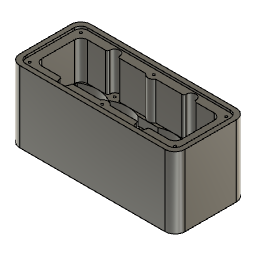
Main Clock Body (Autodesk Fusion 360 design; units mm, degrees)
Autodesk Fusion 360 part; units mm, degrees
sketch "Main Body" plane through (0, 0, 0) normal (0, 0, 1) x (1, 0, 0)
  line L0 (51, 25) -> (-51, 25)
  line L1 (-58, 18) -> (-58, -18)
  line L2 (-51, -25) -> (51, -25)
  line L3 (58, -18) -> (58, 18)
  line L4 (58, 25) -> (-58, -25) construction
  line L5 (-58, 25) -> (58, -25) construction
  arc A0 (-51, 25) -> (-58, 18) centre (-51, 18) ccw
  arc A1 (-58, -18) -> (-51, -25) centre (-51, -18) ccw
  arc A2 (51, -25) -> (58, -18) centre (51, -18) ccw
  arc A3 (58, 18) -> (51, 25) centre (51, 18) ccw
  line L6 (-50, -21.8) -> (50, -21.8)
  line L7 (-54.8, -21.8) -> (54.8, 21.8) construction
  line L8 (54.8, -21.8) -> (-54.8, 21.8) construction
  line L9 (-50, -21.8) -> (50, -21.8)
  line L10 (-50, -21.8) -> (50, -21.8)
  dimension "d1" = 116
  dimension "d2" = 50
  dimension "d3" = 7
  dimension "d4" = 7
  dimension "d5" = 7
  dimension "d6" = 7
  constraint perpendicular L0 L1
  constraint parallel L0 L2
  constraint parallel L1 L3
  constraint horizontal L0
  constraint coincident L4 origin
  constraint coincident L5 origin
  constraint coincident L5.start L0
  constraint coincident L5.start L1
  constraint tangent L0 A0
  constraint tangent L1 A0
  constraint coincident L4.end L1
  constraint coincident L4.end L2
  constraint tangent L1 A1
  constraint tangent L2 A1
  constraint coincident L5.end L2
  constraint coincident L5.end L3
  constraint tangent L2 A2
  constraint tangent L3 A2
  constraint coincident L4.start L3
  constraint coincident L4.start L0
  constraint tangent L3 A3
  constraint tangent L0 A3
  measures "d1" distance of L4.end L5.end
  measures "d2" distance of L5.start L4.end
  measures "d3" radius of A0
  measures "d4" radius of A1
  measures "d5" radius of A2
  measures "d6" radius of A3
  measures "d10" distance of L8.start
extrude "Extrude1" add sketch "Main Body" along normal blind 50
sketch "Back Panel" plane through (0, 0, 50) normal (0, 0, 1) x (-1, 0, 0)
  arc A0 (-58, -18) -> (-51, -25) centre (-51, -18) ccw
  line L0 (-51, -25) -> (51, -25)
  arc A1 (51, -25) -> (58, -18) centre (51, -18) ccw
  line L1 (58, -18) -> (58, 18)
  arc A2 (58, 18) -> (51, 25) centre (51, 18) ccw
  line L2 (51, 25) -> (-51, 25)
  arc A3 (-51, 25) -> (-58, 18) centre (-51, 18) ccw
  line L3 (-58, 18) -> (-58, -18)
  line L4 (-50, -21.8) -> (50, -21.8)
  line L5 (54.8, -17) -> (54.8, 17)
  line L6 (50, 21.8) -> (-50, 21.8)
  line L7 (-54.8, 17) -> (-54.8, -17)
  line L8 (-54.8, -21.8) -> (54.8, 21.8) construction
  line L9 (54.8, -21.8) -> (-54.8, 21.8) construction
  arc A4 (50, -21.8) -> (54.8, -17) centre (50, -17) ccw
  arc A5 (54.8, 17) -> (50, 21.8) centre (50, 17) ccw
  arc A6 (-50, 21.8) -> (-54.8, 17) centre (-50, 17) ccw
  arc A7 (-54.8, -17) -> (-50, -21.8) centre (-50, -17) ccw
  dimension "d9" = 109.6
  dimension "d10" = 43.6
  dimension "d11" = 4.8
  dimension "d12" = 4.8
  dimension "d13" = 4.8
  dimension "d14" = 4.8
  constraint perpendicular L4 L5
  constraint parallel L4 L6
  constraint parallel L5 L7
  constraint horizontal L4
  constraint coincident L8 origin
  constraint coincident L9 origin
  constraint coincident L9.start L4
  constraint coincident L9.start L5
  constraint tangent L4 A4
  constraint tangent L5 A4
  constraint coincident L8.end L5
  constraint coincident L8.end L6
  constraint tangent L5 A5
  constraint tangent L6 A5
  constraint coincident L9.end L6
  constraint coincident L9.end L7
  constraint tangent L6 A6
  constraint tangent L7 A6
  constraint coincident L8.start L7
  constraint coincident L8.start L4
  constraint tangent L7 A7
  constraint tangent L4 A7
  measures "d9" distance of L8.end L9.end
  measures "d10" distance of L9.start L8.end
  measures "d11" radius of A4
  measures "d12" radius of A5
  measures "d13" radius of A6
  measures "d14" radius of A7
extrude "Extrude2" cut sketch "Back Panel" against normal blind 1.6 contours L4 L5 L6 L7 A4 A5 A6 A7
sketch "Electronics Cavity" plane through (0, 0, 48.4) normal (0, 0, 1) x (-1, 0, 0)
  arc A0 (-54.8, -17) -> (-50, -21.8) centre (-50, -17) ccw
  line L0 (-50, -21.8) -> (50, -21.8)
  arc A1 (50, -21.8) -> (54.8, -17) centre (50, -17) ccw
  line L1 (54.8, -17) -> (54.8, 17)
  arc A2 (54.8, 17) -> (50, 21.8) centre (50, 17) ccw
  line L2 (50, 21.8) -> (-50, 21.8)
  arc A3 (-50, 21.8) -> (-54.8, 17) centre (-50, 17) ccw
  line L3 (-54.8, 17) -> (-54.8, -17)
  line L4 (49, 11.5) -> (49, -11.5)
  line L5 (-49, -11.5) -> (-49, 11.5)
  arc A4 (44.5, -16) -> (49, -11.5) centre (44.5, -11.5) ccw
  arc A5 (49, 11.5) -> (44.5, 16) centre (44.5, 11.5) ccw
  arc A6 (-44.5, 16) -> (-49, 11.5) centre (-44.5, 11.5) ccw
  arc A7 (-49, -11.5) -> (-44.5, -16) centre (-44.5, -11.5) ccw
  line L6 (44.5, -16) -> (31.75, -16)
  line L7 (-31.75, -16) -> (-44.5, -16)
  line L8 (31.75, 16) -> (44.5, 16)
  line L9 (-44.5, 16) -> (-31.75, 16)
  arc A8 (-3.4641, 16) -> (3.4641, 16) centre (0, 18) ccw
  line L10 (-3.4641, -16) -> (-21.75, -16)
  line L11 (-21.75, 16) -> (-3.4641, 16)
  line L12 (3.4641, 16) -> (21.75, 16)
  line L13 (26.75, 0) -> (-26.75, 0) construction
  line L14 (26.75, -17.5) -> (26.75, 17.5) construction
  line L15 (-26.75, -17.5) -> (-26.75, 17.5) construction
  line L16 (0, 18) -> (0, -18) construction
  arc A9 (3.4641, -16) -> (-3.4641, -16) centre (0, -18) ccw
  line L17 (49, 0) -> (-49, 0) construction
  arc A10 (23.25, -17.5) -> (30.25, -17.5) centre (26.75, -17.5) ccw
  line L18 (26.75, -17.5) -> (23.25, -17.5) construction
  line L19 (26.75, -17.5) -> (30.25, -17.5) construction
  arc A11 (31.75, -16) -> (30.25, -17.5) centre (31.75, -17.5) ccw
  line L20 (31.75, -17.5) -> (31.75, -16) construction
  line L21 (31.75, -17.5) -> (30.25, -17.5) construction
  line L22 (21.75, -16) -> (3.4641, -16)
  arc A12 (23.25, -17.5) -> (21.75, -16) centre (21.75, -17.5) ccw
  line L23 (21.75, -17.5) -> (23.25, -17.5) construction
  line L24 (21.75, -17.5) -> (21.75, -16) construction
  arc A13 (30.25, 17.5) -> (23.25, 17.5) centre (26.75, 17.5) ccw
  line L25 (26.75, 17.5) -> (30.25, 17.5) construction
  line L26 (26.75, 17.5) -> (23.25, 17.5) construction
  arc A14 (30.25, 17.5) -> (31.75, 16) centre (31.75, 17.5) ccw
  line L27 (31.75, 17.5) -> (30.25, 17.5) construction
  line L28 (31.75, 17.5) -> (31.75, 16) construction
  arc A15 (21.75, 16) -> (23.25, 17.5) centre (21.75, 17.5) ccw
  line L29 (21.75, 17.5) -> (21.75, 16) construction
  line L30 (21.75, 17.5) -> (23.25, 17.5) construction
  arc A16 (-23.25, 17.5) -> (-30.25, 17.5) centre (-26.75, 17.5) ccw
  line L31 (-26.75, 17.5) -> (-23.25, 17.5) construction
  line L32 (-26.75, 17.5) -> (-30.25, 17.5) construction
  arc A17 (-23.25, 17.5) -> (-21.75, 16) centre (-21.75, 17.5) ccw
  line L33 (-21.75, 17.5) -> (-23.25, 17.5) construction
  line L34 (-21.75, 17.5) -> (-21.75, 16) construction
  arc A18 (-31.75, 16) -> (-30.25, 17.5) centre (-31.75, 17.5) ccw
  line L35 (-31.75, 17.5) -> (-31.75, 16) construction
  line L36 (-31.75, 17.5) -> (-30.25, 17.5) construction
  arc A19 (-30.25, -17.5) -> (-23.25, -17.5) centre (-26.75, -17.5) ccw
  line L37 (-26.75, -17.5) -> (-30.25, -17.5) construction
  line L38 (-26.75, -17.5) -> (-23.25, -17.5) construction
  arc A20 (-21.75, -16) -> (-23.25, -17.5) centre (-21.75, -17.5) ccw
  line L39 (-21.75, -17.5) -> (-21.75, -16) construction
  line L40 (-21.75, -17.5) -> (-23.25, -17.5) construction
  arc A21 (-30.25, -17.5) -> (-31.75, -16) centre (-31.75, -17.5) ccw
  line L41 (-31.75, -17.5) -> (-30.25, -17.5) construction
  line L42 (-31.75, -17.5) -> (-31.75, -16) construction
  dimension "d19" = 4.5
  dimension "d20" = 4.5
  dimension "d21" = 4.5
  dimension "d22" = 4.5
  dimension "d52" = 4
  dimension "d99" = 53.5
  dimension "d102" = 36
  dimension "d103" = 4
  dimension "d104" = 98
  dimension "d106" = 32
  dimension "d109" = 35
  dimension "d110" = 3.5
  dimension "d111" = 180
  dimension "d112" = 90
  dimension "d113" = 90
  dimension "d114" = 3.5
  dimension "d115" = 180
  dimension "d116" = 90
  dimension "d117" = 90
  dimension "d118" = 35
  dimension "d119" = 3.5
  dimension "d120" = 180
  dimension "d121" = 90
  dimension "d122" = 90
  dimension "d123" = 3.5
  dimension "d124" = 180
  dimension "d125" = 90
  dimension "d126" = 90
  constraint parallel L6 L9
  constraint parallel L4 L5
  constraint horizontal L9
  constraint tangent A4 L6
  constraint tangent L4 A4
  constraint tangent A5 L9
  constraint tangent L4 A5
  constraint tangent A6 L9
  constraint tangent L5 A6
  constraint tangent L5 A7
  constraint tangent A7 L6
  constraint coincident L8.start L9
  constraint collinear L8 L9
  constraint coincident L11.start L9
  constraint collinear L9 L11
  constraint coincident A8.end L11
  constraint collinear L11 L12
  constraint horizontal L13
  constraint midpoint origin L13
  constraint vertical L14
  constraint midpoint L13.start L14
  constraint vertical L15
  constraint midpoint L13.end L15
  constraint vertical L16
  constraint midpoint origin L16
  constraint coincident L16.end A9.centre
  constraint coincident L10.start A9.end
  constraint horizontal L17
  constraint midpoint origin L17
  constraint coincident L4 L17.start
  constraint coincident L5 L17.end
  constraint vertical L4
  constraint midpoint L4 L17.start
  constraint coincident A8.centre L16.start
  constraint coincident L14.start A10.centre
  constraint horizontal L19
  constraint horizontal L21
  constraint coincident L6.end A11.start
  constraint horizontal L22
  constraint horizontal L23
  constraint coincident L22.start A12.end
  constraint collinear L6 L22
  constraint coincident A9.start L22.end
  constraint coincident L14.end A13.centre
  constraint horizontal L26
  constraint horizontal L27
  constraint coincident L8.start A14.end
  constraint horizontal L30
  constraint coincident L12.end A15.start
  constraint coincident L15.end A16.centre
  constraint horizontal L31
  constraint horizontal L33
  constraint coincident L11.start A17.end
  constraint horizontal L36
  constraint coincident L9.end A18.start
  constraint coincident L15.start A19.centre
  constraint horizontal L38
  constraint horizontal L40
  constraint coincident L10.end A20.start
  constraint collinear L10 L22
  constraint horizontal L41
  constraint coincident L7.start A21.end
  constraint collinear L7 L10
  measures "d19" radius of A4
  measures "d20" radius of A5
  measures "d21" radius of A6
  measures "d22" radius of A7
  measures "d52" radius of A8
  measures "d99" distance of L13.start L13.end
  measures "d102" distance of A8.centre L16.end
  measures "d103" radius of A9
  measures "d104" distance of L17.start L17.end
  measures "d106" distance of A4.start A5.end
  measures "d109" distance of L14.start L14.end
  measures "d110" radius of A10
  measures "d111" angle of L18 L19
  measures "d112" angle of L20 L21
  measures "d113" angle of L23 L24
  measures "d114" radius of A13
  measures "d115" angle of L25 L26
  measures "d116" angle of L27 L28
  measures "d117" angle of L29 L30
  measures "d118" distance of L15.start L15.end
  measures "d119" radius of A16
  measures "d120" angle of L31 L32
  measures "d121" angle of L33 L34
  measures "d122" angle of L35 L36
  measures "d123" radius of A19
  measures "d124" angle of L37 L38
  measures "d125" angle of L39 L40
  measures "d126" angle of L41 L42
extrude "Extrude3" cut sketch "Electronics Cavity" against normal blind 26.6 contours L4 L5 A4 A5 A6 A7 L6 L7 L8 L9 A8 L10 L11 L12 A9 A10 A11 L22 A12 A13 A14 A15 A16 A17 A18 A19 A20 A21
sketch "Tube Cavities" plane through (0, 0, 21.8) normal (0, 0, 1) x (-1, 0, 0)
  line L0 (-31.75, 16) -> (-44.5, 16)
  arc A0 (-44.5, 16) -> (-49, 11.5) centre (-44.5, 11.5) ccw
  line L1 (-49, 11.5) -> (-49, -11.5)
  arc A1 (-49, -11.5) -> (-44.5, -16) centre (-44.5, -11.5) ccw
  line L2 (-44.5, -16) -> (-31.75, -16)
  line L3 (31.75, -16) -> (44.5, -16)
  arc A2 (44.5, -16) -> (49, -11.5) centre (44.5, -11.5) ccw
  line L4 (49, -11.5) -> (49, 11.5)
  arc A3 (49, 11.5) -> (44.5, 16) centre (44.5, 11.5) ccw
  line L5 (44.5, 16) -> (31.75, 16)
  line L6 (21.75, 16) -> (3.4641, 16)
  arc A4 (-3.4641, 16) -> (3.4641, 16) centre (0, 18) ccw
  line L7 (16, 0) -> (-16, 0) construction
  line L8 (37.5, 0) -> (-37.5, 0) construction
  line L9 (37.5, -5) -> (37.5, 5) construction
  arc A5 (48.5, 12.8885) -> (27.25, 13.3286) centre (37.5, -5) ccw
  arc A6 (27.25, -13.3286) -> (48.5, -12.8885) centre (37.5, 5) ccw
  line L10 (37.5, -16) -> (37.5, 16) construction
  line L11 (16, -16) -> (16, 16) construction
  line L12 (16, 5) -> (16, -5) construction
  line L13 (37.5, 0) -> (48.5, 0) construction
  line L14 (48.5, -12.8885) -> (48.5, 12.8885)
  line L15 (27.25, -13.3286) -> (26.25, -13.3286)
  line L16 (27.25, 13.3286) -> (26.25, 13.3286)
  arc A7 (5, -12.8885) -> (26.25, -13.3286) centre (16, 5) ccw
  arc A8 (26.25, 13.3286) -> (5, 12.8885) centre (16, -5) ccw
  line L17 (5, -12.8885) -> (5, 12.8885)
  line L18 (16, 0) -> (5, 0) construction
  line L19 (-16, -5) -> (-16, 5) construction
  line L20 (-16, -16) -> (-16, 16) construction
  line L21 (-16, 0) -> (-5, 0) construction
  line L22 (-37.5, -5) -> (-37.5, 5) construction
  line L23 (-37.5, -16) -> (-37.5, 16) construction
  arc A9 (-48.5, -12.8885) -> (-27.25, -13.3286) centre (-37.5, 5) ccw
  arc A10 (-26.25, -13.3286) -> (-5, -12.8885) centre (-16, 5) ccw
  arc A11 (-5, 12.8885) -> (-26.25, 13.3286) centre (-16, -5) ccw
  arc A12 (-27.25, 13.3286) -> (-48.5, 12.8885) centre (-37.5, -5) ccw
  line L24 (-5, -12.8885) -> (-5, 12.8885)
  line L25 (-48.5, -12.8885) -> (-48.5, 12.8885)
  line L26 (-26.25, -13.3286) -> (-27.25, -13.3286)
  line L27 (-26.25, 13.3286) -> (-27.25, 13.3286)
  line L28 (-37.5, 0) -> (-48.5, 0) construction
  arc A13 (3.4641, -16) -> (-3.4641, -16) centre (0, -18) ccw
  arc A14 (23.25, -17.5) -> (30.25, -17.5) centre (26.75, -17.5) ccw
  arc A15 (31.75, -16) -> (30.25, -17.5) centre (31.75, -17.5) ccw
  arc A16 (30.25, 17.5) -> (31.75, 16) centre (31.75, 17.5) ccw
  arc A17 (30.25, 17.5) -> (23.25, 17.5) centre (26.75, 17.5) ccw
  arc A18 (21.75, 16) -> (23.25, 17.5) centre (21.75, 17.5) ccw
  line L29 (-3.4641, 16) -> (-21.75, 16)
  arc A19 (-23.25, 17.5) -> (-21.75, 16) centre (-21.75, 17.5) ccw
  arc A20 (-23.25, 17.5) -> (-30.25, 17.5) centre (-26.75, 17.5) ccw
  arc A21 (-31.75, 16) -> (-30.25, 17.5) centre (-31.75, 17.5) ccw
  arc A22 (-30.25, -17.5) -> (-31.75, -16) centre (-31.75, -17.5) ccw
  arc A23 (-30.25, -17.5) -> (-23.25, -17.5) centre (-26.75, -17.5) ccw
  arc A24 (-21.75, -16) -> (-23.25, -17.5) centre (-21.75, -17.5) ccw
  line L30 (-21.75, -16) -> (-3.4641, -16)
  line L31 (3.4641, -16) -> (21.75, -16)
  arc A25 (23.25, -17.5) -> (21.75, -16) centre (21.75, -17.5) ccw
  point P0 (37.5, 0)
  dimension "d54" = 32
  dimension "d55" = 75
  dimension "d58" = 10
  dimension "d59" = 32
  dimension "d60" = 32
  dimension "d61" = 10
  dimension "d62" = 11
  dimension "d63" = 11
  dimension "d64" = 1
  dimension "d65" = 1
  dimension "d66" = 10
  dimension "d67" = 32
  dimension "d68" = 11
  dimension "d69" = 10
  dimension "d71" = 32
  dimension "d72" = 1
  dimension "d73" = 1
  dimension "d74" = 11
  constraint horizontal L7
  constraint midpoint origin L7
  constraint horizontal L8
  constraint midpoint origin L8
  constraint coincident P0 L8.start
  constraint perpendicular L8 L9
  constraint midpoint P0 L9
  constraint coincident L9.start A5.centre
  constraint coincident L9.end A6.centre
  constraint vertical L10
  constraint midpoint P0 L10
  constraint coincident A6 L10.start
  constraint coincident A5 L10.end
  constraint vertical L11
  constraint midpoint L7.start L11
  constraint vertical L12
  constraint midpoint L7.start L12
  constraint vertical L14
  constraint coincident L13.end L14
  constraint horizontal L13
  constraint horizontal L15
  constraint perpendicular L11 L16
  constraint coincident L12.start A7.centre
  constraint coincident L12.end A8.centre
  constraint vertical L17
  constraint perpendicular L12 L18
  constraint coincident L17 L18.end
  constraint coincident L11.start A7
  constraint coincident L11.end A8
  constraint vertical L19
  constraint midpoint L7.end L19
  constraint vertical L20
  constraint midpoint L7.end L20
  constraint perpendicular L20 L21
  constraint vertical L22
  constraint vertical L23
  constraint midpoint L8.end L23
  constraint midpoint L8.end L22
  constraint coincident L22.end A9.centre
  constraint coincident L23.start A9
  constraint coincident L19.end A10.centre
  constraint coincident L19.start A11.centre
  constraint coincident L22.start A12.centre
  constraint coincident L23.end A12
  constraint coincident L20.end A11
  constraint coincident L20.start A10
  constraint horizontal L26
  constraint horizontal L27
  constraint vertical L25
  constraint vertical L24
  constraint perpendicular L25 L28
  constraint coincident L25 L28.end
  constraint coincident L21.end L24
  measures "d54" distance of L7.start L7.end
  measures "d55" distance of P0 L8.end
  measures "d58" distance of L9.start L9.end
  measures "d59" distance of L10.start L10.end
  measures "d60" distance of L11.start L11.end
  measures "d61" distance of L12.start L12.end
  measures "d62" distance of P0 L13.end
  measures "d63" distance of L7.start L18.end
  measures "d64" distance of A5.end L16.end
  measures "d65" distance of A6.start L15.end
  measures "d66" distance of L19.start L19.end
  measures "d67" distance of L20.start L20.end
  measures "d68" distance of L7.end L21.end
  measures "d69" distance of L22.start L22.end
  measures "d71" distance of L23.start L23.end
  measures "d72" distance of A9.end A10.start
  measures "d73" distance of A11.end A12.start
  measures "d74" distance of L8.end L28.end
extrude "Extrude4" cut sketch "Tube Cavities" against normal blind 23.4 contours A9 A10 A11 A12 L24 L25 L26 L27 | A5 A6 L14 L15 L16 A7 A8 L17
sketch "Electronics Cavity Extension" plane through (0, 0, 21.8) normal (0, 0, 1) x (-1, 0, 0)
  arc A0 (-5, 12.8885) -> (-16, 16) centre (-16, -5) ccw
  line L0 (-5, 12.8885) -> (-5, -12.8885)
  arc A1 (-16, -16) -> (-5, -12.8885) centre (-16, 5) ccw
  arc A2 (5, -12.8885) -> (16, -16) centre (16, 5) ccw
  line L1 (5, -12.8885) -> (5, 12.8885)
  arc A3 (16, 16) -> (5, 12.8885) centre (16, -5) ccw
  line L2 (16, 16) -> (3.4641, 16)
  arc A4 (-3.4641, 16) -> (3.4641, 16) centre (0, 18) ccw
  line L3 (-7.0557, -14) -> (7.0557, -14)
  line L4 (7.0557, -14) -> (7.0557, 14)
  line L5 (7.0557, 14) -> (-7.0557, 14)
  line L6 (-7.0557, 14) -> (-7.0557, -14)
  line L7 (-7.0557, -14) -> (7.0557, 14) construction
  line L8 (7.0557, -14) -> (-7.0557, 14) construction
  arc A5 (3.4641, -16) -> (-3.4641, -16) centre (0, -18) ccw
  line L9 (-3.4641, 16) -> (-16, 16)
  line L10 (-16, -16) -> (-3.4641, -16)
  line L11 (3.4641, -16) -> (16, -16)
  point P0 (0, -14)
  constraint perpendicular L3 L4
  constraint parallel L3 L5
  constraint parallel L4 L6
  constraint horizontal L3
  constraint coincident L7 origin
  constraint coincident L8 origin
  constraint coincident A1 L3.start
  constraint midpoint A5 P0
  constraint coincident L3 P0
extrude "Extrude5" cut sketch "Electronics Cavity Extension" against normal blind 6 contours A0 L0 A1 A2 L1 A3 L3 L5
sketch "Back Cover Drills" plane through (0, 0, 48.4) normal (0, 0, 1) x (-1, 0, 0)
  line L0 (31.75, 16) -> (44.5, 16)
  arc A0 (49, 11.5) -> (44.5, 16) centre (44.5, 11.5) ccw
  line L1 (49, 11.5) -> (49, -11.5)
  arc A1 (44.5, -16) -> (49, -11.5) centre (44.5, -11.5) ccw
  line L2 (-3.4641, -16) -> (-21.75, -16)
  line L3 (-31.75, -16) -> (-44.5, -16)
  arc A2 (-49, -11.5) -> (-44.5, -16) centre (-44.5, -11.5) ccw
  line L4 (-49, -11.5) -> (-49, 11.5)
  arc A3 (-44.5, 16) -> (-49, 11.5) centre (-44.5, 11.5) ccw
  line L5 (-44.5, 16) -> (-31.75, 16)
  arc A4 (-54.8, -17) -> (-50, -21.8) centre (-50, -17) ccw
  line L6 (-50, -21.8) -> (50, -21.8)
  arc A5 (50, -21.8) -> (54.8, -17) centre (50, -17) ccw
  line L7 (54.8, -17) -> (54.8, 17)
  arc A6 (54.8, 17) -> (50, 21.8) centre (50, 17) ccw
  line L8 (50, 21.8) -> (-50, 21.8)
  arc A7 (-50, 21.8) -> (-54.8, 17) centre (-50, 17) ccw
  line L9 (-54.8, 17) -> (-54.8, -17)
  line L10 (0, -18) -> (0, 18) construction
  line L11 (51, -18) -> (-51, -18) construction
  line L12 (51, 18) -> (-51, 18) construction
  circle A8 centre (51, 18) radius 0.795
  circle A9 centre (51, -18) radius 0.795
  circle A10 centre (0, -18) radius 0.795
  circle A11 centre (0, 18) radius 0.795
  circle A12 centre (-51, 18) radius 0.795
  circle A13 centre (-51, -18) radius 0.795
  arc A14 (3.4641, -16) -> (-3.4641, -16) centre (0, -18) ccw
  line L13 (-21.75, 16) -> (-3.4641, 16)
  arc A15 (-3.4641, 16) -> (3.4641, 16) centre (0, 18) ccw
  line L14 (3.4641, 16) -> (21.75, 16)
  arc A16 (31.75, -16) -> (30.25, -17.5) centre (31.75, -17.5) ccw
  arc A17 (23.25, -17.5) -> (30.25, -17.5) centre (26.75, -17.5) ccw
  arc A18 (23.25, -17.5) -> (21.75, -16) centre (21.75, -17.5) ccw
  line L15 (21.75, -16) -> (3.4641, -16)
  arc A19 (-21.75, -16) -> (-23.25, -17.5) centre (-21.75, -17.5) ccw
  arc A20 (-30.25, -17.5) -> (-23.25, -17.5) centre (-26.75, -17.5) ccw
  arc A21 (-30.25, -17.5) -> (-31.75, -16) centre (-31.75, -17.5) ccw
  arc A22 (-31.75, 16) -> (-30.25, 17.5) centre (-31.75, 17.5) ccw
  arc A23 (-23.25, 17.5) -> (-30.25, 17.5) centre (-26.75, 17.5) ccw
  arc A24 (-23.25, 17.5) -> (-21.75, 16) centre (-21.75, 17.5) ccw
  arc A25 (21.75, 16) -> (23.25, 17.5) centre (21.75, 17.5) ccw
  arc A26 (30.25, 17.5) -> (23.25, 17.5) centre (26.75, 17.5) ccw
  arc A27 (30.25, 17.5) -> (31.75, 16) centre (31.75, 17.5) ccw
  line L16 (44.5, -16) -> (31.75, -16)
  dimension "d79" = 36
  dimension "d80" = 102
  dimension "d81" = 102
  dimension "d82" = 1.59
  dimension "d83" = 1.59
  dimension "d84" = 1.59
  dimension "d85" = 1.59
  dimension "d86" = 1.59
  dimension "d87" = 1.59
  constraint vertical L10
  constraint midpoint origin L10
  constraint horizontal L11
  constraint midpoint L10.start L11
  constraint horizontal L12
  constraint midpoint L10.end L12
  constraint coincident L12.start A8.centre
  constraint coincident L11.start A9.centre
  constraint coincident L10.start A10.centre
  constraint coincident L10.end A11.centre
  constraint coincident L12.end A12.centre
  constraint coincident L11.end A13.centre
  measures "d79" distance of L10.start L10.end
  measures "d80" distance of L11.start L11.end
  measures "d81" distance of L12.start L12.end
  measures "d82" diameter of A8
  measures "d83" diameter of A9
  measures "d84" diameter of A10
  measures "d85" diameter of A11
  measures "d86" diameter of A12
  measures "d87" diameter of A13
extrude "Extrude6" cut sketch "Back Cover Drills" against normal blind 10 contours A8 | A9 | A10 | A11 | A12 | A13
sketch "PCB Drills" plane through (0, 0, 21.8) normal (0, 0, 1) x (-1, 0, 0)
  arc A0 (27.25, -13.3286) -> (37.5, -16) centre (37.5, 5) ccw
  line L0 (27.25, -13.3286) -> (26.25, -13.3286)
  arc A1 (16, -16) -> (26.25, -13.3286) centre (16, 5) ccw
  line L1 (26.75, 0) -> (-26.75, 0) construction
  line L2 (26.75, -17.5) -> (26.75, 17.5) construction
  line L3 (-26.75, -17.5) -> (-26.75, 17.5) construction
  circle A2 centre (26.75, -17.5) radius 0.795
  circle A3 centre (26.75, 17.5) radius 0.795
  circle A4 centre (-26.75, -17.5) radius 0.795
  circle A5 centre (-26.75, 17.5) radius 0.795
  line L4 (31.75, -16) -> (37.5, -16)
  line L5 (16, -16) -> (21.75, -16)
  arc A6 (23.25, -17.5) -> (21.75, -16) centre (21.75, -17.5) ccw
  arc A7 (23.25, -17.5) -> (30.25, -17.5) centre (26.75, -17.5) ccw
  arc A8 (31.75, -16) -> (30.25, -17.5) centre (31.75, -17.5) ccw
  dimension "d90" = 53.5
  dimension "d91" = 35
  dimension "d92" = 35
  dimension "d93" = 1.59
  dimension "d94" = 1.59
  dimension "d95" = 1.59
  dimension "d96" = 1.59
  constraint horizontal L1
  constraint midpoint origin L1
  constraint vertical L2
  constraint midpoint L1.start L2
  constraint vertical L3
  constraint midpoint L1.end L3
  constraint coincident L2.end A3.centre
  constraint coincident L3.start A4.centre
  constraint coincident L3.end A5.centre
  constraint coincident L2.start A2.centre
  measures "d90" distance of L1.start L1.end
  measures "d91" distance of L2.start L2.end
  measures "d92" distance of L3.start L3.end
  measures "d93" diameter of A2
  measures "d94" diameter of A3
  measures "d95" diameter of A4
  measures "d96" diameter of A5
extrude "Extrude7" cut sketch "PCB Drills" against normal blind 10 contours A2 | A3 | A4 | A5
